nixal_reprap_XidlerComparible_robust (Autodesk Fusion 360 design; units mm, degrees)
Autodesk Fusion 360 part; units mm, degrees
sketch "Sketch1" plane through (0, 0, 0) normal (0, 1, 0) x (1, 0, 0)
  circle A0 centre (0, 0) radius 4
  circle A1 centre (21, -2) radius 4
  circle A2 centre (21, -2) radius 13
  circle A3 centre (21, -2) radius 8 construction
  circle A4 centre (13, -1.9989) radius 1.8
  circle A5 centre (29, -2.0036) radius 1.8
  line L0 (21, -2) -> (21, 11) construction
  line L1 (21, -2) -> (34, -2) construction
  line L2 (41, 31) -> (-24, 31)
  line L3 (41, 31) -> (41, -15)
  circle A6 centre (0, 0) radius 10.5
  circle A7 centre (0, 0) radius 13.5
  line L4 (40.8669, 9) -> (-49.1331, 9)
  line L5 (-49.1331, 9) -> (-49.1331, 26)
  line L6 (-49.1331, 26) -> (40.8669, 26)
  line L7 (40.8669, 26) -> (40.8669, 9)
  line L8 (-13.5, 0) -> (-13.5, 9)
  line L9 (34, -2) -> (34, 9)
  line L10 (0, 0) -> (9.5068, -9.5849)
  line L11 (0, 0) -> (7.6248, -11.8995)
  circle A8 centre (21, -2) radius 5.5
  line L12 (13.3463, 2.0311) -> (12.2858, 9)
  line L13 (9.5068, -9.5849) -> (14.0455, -12.9834)
  circle A9 centre (21, 6) radius 1.8
  circle A10 centre (20.9776, -10) radius 1.8
  circle A11 centre (21, -2) radius 12.6491
  circle A12 centre (0, 0) radius 13.0384
  circle A13 centre (21, -2) radius 5.25
  line L14 (-48.7267, 25.5998) -> (-9.6603, 25.5998)
  line L15 (-9.6603, 25.5998) -> (-9.6603, 9.5175)
  line L16 (-9.6603, 9.5175) -> (-48.7267, 9.5175)
  line L17 (-48.7267, 9.5175) -> (-48.7267, 25.5998)
  line L18 (-9.2762, 9) -> (-9.2762, 26)
  circle A14 centre (0, 0) radius 10.9156
  line L19 (-48.7267, 18.529) -> (-9.6603, 18.529)
  line L20 (-48.7267, 17.955) -> (-9.6603, 17.955)
  circle A15 centre (0, 0) radius 8
  dimension "d1" = 8
  dimension "d2" = 8
  dimension "d23" = 26
  dimension "d104" = 16
  dimension "d107" = 3.6
  dimension "d108" = 3.6
  dimension "d134" = 33
  dimension "d136" = 31
  dimension "d137" = 20
  dimension "d138" = 41
  dimension "d139" = 21
  dimension "d140" = 27
  dimension "d141" = 17
  dimension "d142" = 90
  dimension "d143" = 5
  dimension "d146" = 11
  dimension "d203" = 3.6
  dimension "d204" = 3.6
  dimension "d211" = 90
  dimension "d225" = 10.5
  dimension "d238" = 16
  constraint coincident A0.centre A6.centre
  constraint concentric A1 A2
  constraint coincident A3 A0.centre
  constraint coincident A3
  constraint coincident A2 A0.centre
  constraint vertical L0
  constraint horizontal L1
  constraint horizontal L2
  constraint vertical L3
  constraint concentric A0 A6
  constraint concentric A6 A7
  constraint horizontal L4
  constraint vertical L5
  constraint horizontal L6
  constraint vertical L7
  constraint coincident A7 A0.centre
  constraint coincident L4
  constraint tangent A7 L8
  constraint tangent A2 L9
  constraint coincident A7
  constraint concentric A3 A8
  constraint tangent A7 L12
  constraint coincident A2
  constraint coincident L0 A0.centre
  constraint concentric A1 A11
  constraint concentric A11 A13
  constraint horizontal L14
  constraint vertical L15
  constraint horizontal L16
  constraint vertical L17
  constraint coincident L6
  constraint perpendicular L6 L18
  constraint concentric A12 A14
  constraint coincident L17
  constraint coincident L15
  constraint perpendicular L15 L19
  constraint perpendicular L15 L20
  measures "d1" diameter of A0
  measures "d2" diameter of A1
  measures "d23" diameter of A2
  measures "d104" diameter of A3
  measures "d107" diameter of A4
  measures "d108" diameter of A5
  measures "d134" distance of A0.centre L2
  measures "d136" distance of A0.centre L2
  measures "d137" distance of A0.centre L3
  measures "d138" distance of A0.centre L3
  measures "d139" diameter of A6
  measures "d140" diameter of A7
  measures "d143" distance of L2 L6
  measures "d146" diameter of A8
  measures "d203" diameter of A9
  measures "d204" diameter of A10
  measures "d211" angle of L4 L8
  measures "d225" diameter of A13
  measures "d238" diameter of A15
extrude "Extrude24" add sketch "Sketch1" along normal blind 62 contours A6 L4 L11 A14 | A6 L10 L11 A14 | A2 A6 L10 A14 | A6 L4 A14 | L10 L11 A12 A14 | L4 L11 A12 A14 | A2 A6 A11 A14 | A2 L10 A12 A14 | A2 A6 L4 A14 | L4 A12 L18 A14 | A7 L10 L11 A12 | A7 L4 L11 A12 | A2 A6 A11 A14 | A2 A11 A12 A14 | A6 A11 A14 | A2 A7 L10 A12 | A2 L4 A12 A14 | L4 A12 L18 | A7 L4 A12 L18 | A2 A11 A12 A14 | A2 A7 A11 A12 | A4 A11 A12 A14 | A7 L4 A12 L18 | A2 A7 L4 A12 | A7 L4 L8 | A7 L4 L5 L6 L18 | A2 A7 A11 A12 | A4 A7 A11 A12 | A2 A7 L4 L12 | A2 A7 L4 L6 L7 L18 | A2 A7 L12 A11 | A4 A7 A11 A12 | A4 A7 A12 | A4 A12 | A7 L12 A11 | A2 L4 A11 | L4 A11 | L14 L15 L17 L19 | L15 L17 L19 L20 | L15 L16 L17 L20 makes body 1
extrude "Extrude26" add sketch "Sketch1" along normal blind 62 and the other way blind -54 contours A2 A7 L13 | A2 A7 L4 L13 A11 | A4 A7 L4 L12 A11 | A2 L4 L12 | A2 L4 L12 A11 | A2 L4 L9 bodies 1
sketch "Sketch7" plane through (40.8669, 0, 0) normal (1, 0, 0) x (0, 0, -1)
  line L0 (9, 0) -> (26, 0)
  line L1 (26, 0) -> (26, 62)
  line L2 (26, 62) -> (9, 62)
  line L3 (9, 62) -> (9, 0)
  line L4 (9, 62) -> (26, 0) construction
  line L5 (9, 0) -> (26, 62) construction
  line L6 (17.5, 31) -> (17.5, 53.5) construction
  line L7 (17.5, 31) -> (17.5, 8.5) construction
  circle A0 centre (17.5, 53.5) radius 6
  circle A1 centre (17.5, 8.5) radius 6
  line L8 (23, 46) -> (12, 46)
  line L9 (12, 46) -> (12, 16)
  line L10 (12, 16) -> (23, 16)
  line L11 (23, 16) -> (23, 46)
  line L12 (23, 46) -> (12, 16) construction
  line L13 (12, 46) -> (23, 16) construction
  line L14 (22.7211, 43.5) -> (12.2789, 43.5)
  line L15 (12.2789, 43.5) -> (12.2789, 18.5)
  line L16 (12.2789, 18.5) -> (22.7211, 18.5)
  line L17 (22.7211, 18.5) -> (22.7211, 43.5)
  line L18 (22.7211, 43.5) -> (12.2789, 18.5) construction
  line L19 (12.2789, 43.5) -> (22.7211, 18.5) construction
  line L20 (9, 69.9847) -> (26, 69.9847)
  line L21 (26, 69.9847) -> (26, -8.2428)
  line L22 (26, -8.2428) -> (9, -8.2428)
  line L23 (9, -8.2428) -> (9, 69.9847)
  line L24 (15.7453, 69.9847) -> (18.9725, 69.9847)
  line L25 (18.9725, 69.9847) -> (18.9725, 53.5)
  line L26 (18.9725, 53.5) -> (15.7453, 53.5)
  line L27 (15.7453, 53.5) -> (15.7453, 69.9847)
  line L28 (15.6365, -8.2428) -> (19, -8.2428)
  line L29 (19, -8.2428) -> (19, 8)
  line L30 (19, 8) -> (15.6365, 8)
  line L31 (15.6365, 8) -> (15.6365, -8.2428)
  dimension "d173" = 22.5
  dimension "d174" = 22.5
  dimension "d175" = 12
  dimension "d176" = 12
  dimension "d179" = 30
  dimension "d180" = 11
  dimension "d195" = 25
  constraint midpoint L4
  constraint perpendicular L8 L9
  constraint parallel L8 L10
  constraint parallel L9 L11
  constraint horizontal L8
  constraint coincident L12
  constraint coincident L13
  constraint perpendicular L14 L15
  constraint parallel L14 L16
  constraint parallel L15 L17
  constraint horizontal L14
  constraint coincident L18
  constraint coincident L19
  constraint horizontal L20
  constraint vertical L21
  constraint horizontal L22
  constraint vertical L23
  constraint horizontal L24
  constraint vertical L25
  constraint horizontal L26
  constraint vertical L27
  constraint coincident L20 origin
  constraint horizontal L28
  constraint vertical L29
  constraint horizontal L30
  constraint vertical L31
  constraint coincident L22 origin
  measures "d174" distance of origin
  measures "d175" diameter of A0
  measures "d176" diameter of A1
  measures "d179" distance of origin
  measures "d195" distance of origin
extrude "Extrude27" cut sketch "Sketch7" against normal blind 100 contours A1 L29 L30 L31 | A1 L29 L30 L31 | A0 L25 L26 L27 | A0 L25 L26 L27 bodies 1
extrude "Extrude28" cut sketch "Sketch7" against normal blind 52 contours L8 L9 L10 L11 | L14 L15 L16 L17 bodies 1
sketch "Sketch8" plane through (0, 0, -9) normal (0, 0, 1) x (1, 0, 0)
  line L0 (-49.1331, 0) -> (-13.5, 0)
  line L1 (-13.5, 0) -> (-13.5, 62)
  line L2 (-13.5, 62) -> (-49.1331, 62)
  line L3 (-49.1331, 62) -> (-49.1331, 0)
  line L4 (-49.1331, 62) -> (-13.5, 0) construction
  line L5 (-13.5, 62) -> (-49.1331, 0) construction
  circle A0 centre (-31.3165, 31) radius 15
  line L6 (-15.8165, 47) -> (-46.8165, 47) construction
  line L7 (-46.8165, 47) -> (-46.8165, 15) construction
  line L8 (-46.8165, 15) -> (-15.8165, 15) construction
  line L9 (-15.8165, 15) -> (-15.8165, 47) construction
  line L10 (-15.8165, 47) -> (-46.8165, 15) construction
  line L11 (-46.8165, 47) -> (-15.8165, 15) construction
  circle A1 centre (-46.8165, 47) radius 1.65
  circle A2 centre (-15.8165, 47) radius 1.65
  circle A3 centre (-46.8165, 15) radius 1.65
  circle A4 centre (-15.8165, 15) radius 1.65
  circle A5 centre (-46.8165, 47) radius 3
  circle A6 centre (-15.8165, 47) radius 3
  circle A7 centre (-15.8165, 15) radius 3
  line L12 (-49.1331, 38.5778) -> (-44.2617, 38.5778)
  line L13 (-24.2799, 0) -> (-24.2799, 17.7529)
  line L14 (-49.1331, 62) -> (-13.5, 62)
  line L15 (-13.5, 62) -> (-13.5, 0)
  line L16 (-13.5, 0) -> (-49.1331, 0)
  line L17 (-49.1331, 0) -> (-49.1331, 62)
  arc A8 (-44.1331, 62) -> (-49.1331, 57) centre (-44.1331, 57) ccw
  line L18 (-49.1331, 62) -> (-13.5, 62)
  line L19 (-13.5, 62) -> (-13.5, 70.2436)
  line L20 (-13.5, 70.2436) -> (-49.1331, 70.2436)
  line L21 (-49.1331, 70.2436) -> (-49.1331, 62)
  dimension "d183" = 30
  dimension "d184" = 31
  dimension "d185" = 32
  dimension "d186" = 3.3
  dimension "d187" = 3.3
  dimension "d188" = 3.3
  dimension "d189" = 3.3
  dimension "d190" = 6
  dimension "d191" = 6
  dimension "d192" = 6
  dimension "d202" = 5
  constraint midpoint L4
  constraint perpendicular L6 L7
  constraint parallel L6 L8
  constraint parallel L7 L9
  constraint horizontal L6
  constraint coincident L10
  constraint coincident L11
  constraint concentric A1 A5
  constraint coincident L3 origin
  constraint perpendicular L7 L12
  constraint coincident A0 origin
  constraint perpendicular L8 L13
  constraint horizontal L14
  constraint vertical L15
  constraint horizontal L16
  constraint vertical L17
  constraint coincident L16 origin
  constraint tangent L14 A8
  constraint tangent L17 A8
  constraint coincident L14
  constraint coincident L17
  constraint horizontal L18
  constraint vertical L19
  constraint horizontal L20
  constraint vertical L21
  measures "d183" diameter of A0
  measures "d184" distance of origin
  measures "d186" diameter of A1
  measures "d187" diameter of A2
  measures "d188" diameter of A3
  measures "d189" diameter of A4
  measures "d190" diameter of A5
  measures "d191" diameter of A6
  measures "d192" diameter of A7
  measures "d202" radius of A8
extrude "Extrude29" cut sketch "Sketch8" against normal blind 40 contours L0 L3 A0 L12 L13 L16 L17 | A0 | L2 L3 L14 L17 A8 L18 | A3 bodies 1
extrude "Extrude30" cut sketch "Sketch7" against normal blind 65 contours L14 L15 L16 L17 bodies 1
extrude "Extrude31" cut sketch "Sketch8" against normal blind 40 contours A1 | A2 | A4 bodies 1
extrude "Extrude32" cut sketch "Sketch8" against normal blind 9 contours L3 A5 L17 | L3 A5 L17 | L1 A7 L15 | L1 A7 L15 | L1 A6 L15 | L1 A6 L15 bodies 1
extrude "Extrude33" add sketch "Sketch7" against normal blind 50 contours L0 L22 L23 L31 | L0 L22 L28 L29 L31 | L2 L20 L23 L27 | L0 L21 L22 L29 | L2 L20 L24 L25 L27 | L2 L20 L21 L25 bodies 1
extrude "Extrude34" cut sketch "Sketch7" against normal blind 50 contours L2 L20 L24 L25 L27 | L2 A0 L25 L27 | A0 L25 L26 L27 picked at (17.3571, 55.4994) bodies 1
extrude "Extrude35" cut sketch "Sketch7" against normal blind 50 contours L0 A1 L29 L31 | L0 L22 L28 L29 L31 | A1 L29 L30 L31 picked at (17.3157, 6.1677) bodies 1
extrude "Extrude36" cut sketch "Sketch1" along normal blind 65 contours A6 L10 L11 A14 | L10 L11 A12 A14 | A7 L10 L11 A12 bodies 1
sketch "Sketch9" plane through (0, -8.2428, 0) normal (0, -1, 0) x (1, 0, 0)
  line L0 (-9.1331, -15.6365) -> (40.8669, -15.6365)
  line L1 (40.8669, -15.6365) -> (40.8669, -9)
  line L2 (40.8669, -9) -> (-9.1331, -9)
  line L3 (-9.1331, -9) -> (-9.1331, -15.6365)
  circle A0 centre (0, 0) radius 10.5
  line L4 (40.8669, -9) -> (-49.1331, -9)
extrude "Extrude37" cut sketch "Sketch9" against normal blind 80 contours L2 A0 L4 picked at (1.3817, -9.2157) bodies 1
sketch "Sketch10" plane through (0, 0, -26) normal (0, 0, -1) x (-1, 0, 0)
  circle A0 centre (46.8165, 47) radius 1.65
  circle A1 centre (15.8165, 47) radius 1.65
  circle A2 centre (15.8165, 15) radius 1.65
  arc A3 (49.1331, 57) -> (44.1331, 62) centre (44.1331, 57) ccw
  line L0 (44.1331, 62) -> (9.1331, 62)
  line L1 (9.1331, 62) -> (9.1331, 69.9847)
  line L2 (9.1331, 69.9847) -> (-40.8669, 69.9847)
  line L3 (-40.8669, 69.9847) -> (-40.8669, -8.2428)
  line L4 (-40.8669, -8.2428) -> (9.1331, -8.2428)
  line L5 (9.1331, -8.2428) -> (9.1331, 0)
  line L6 (9.1331, 0) -> (24.2799, 0)
  line L7 (24.2799, 0) -> (24.2799, 17.7529)
  arc A4 (44.2617, 38.5778) -> (24.2799, 17.7529) centre (31.3165, 31) ccw
  line L8 (44.2617, 38.5778) -> (49.1331, 38.5778)
  line L9 (49.1331, 38.5778) -> (49.1331, 57)
  circle A5 centre (-35, 66) radius 1.65
  circle A6 centre (-11, 66) radius 1.65
  circle A7 centre (-11, -4) radius 1.65
  circle A8 centre (-35, -4) radius 1.65
  dimension "d216" = 3.3
  dimension "d217" = 3.3
  dimension "d220" = 3.3
  dimension "d221" = 3.3
  measures "d216" diameter of A5
  measures "d217" diameter of A6
  measures "d220" diameter of A7
  measures "d221" diameter of A8
extrude "Extrude38" cut sketch "Sketch10" against normal blind 31 contours A5 | A6 | A7 | A8 bodies 1
extrude "Extrude39" add sketch "Sketch1" along normal blind 70 and the other way blind -62 separate body contours A7 L10 L11 A12 | A7 L4 L11 A12 | A2 A7 L13 | A2 A7 L4 L13 A11 makes body 2
extrude "Extrude40" add sketch "Sketch1" along normal blind 70 and the other way blind -62 separate body contours A8 makes body 3
extrude "Extrude41" add sketch "Sketch1" along normal blind 70 and the other way blind -62 separate body contours A7 L4 L5 L6 L18 makes body 4
extrude "Extrude42" add sketch "Sketch1" along normal blind 70 and the other way blind -62 separate body contours A6 L4 L11 A14 | A6 L10 L11 A14 | A2 A6 L10 A14 | A6 L4 A14 | A2 A6 A11 A14 | A2 A6 L4 A14 | A2 A6 A11 A14 | A6 A11 A14 makes body 5
extrude "Extrude43" add sketch "Sketch1" along normal blind 70 and the other way blind -62 separate body contours L15 L17 L19 L20 makes body 6
extrude "Extrude44" add sketch "Sketch1" along normal blind 62 contours A2 A6 L4 L10 L11 A15 | A2 A6 A11 | A6 A11 bodies 1 5
extrude "Extrude45" cut sketch "Sketch8" against normal blind 85 contours L0 L1 L2 L3 A0 A5 A6 A7 L12 L13 L14 L15 L16 L17 A8 L18 | L3 A5 L17 | L1 A7 L15 | L1 A6 L15 | L2 L14 L18 L19 L20 L21 picked at (-48.9109, 47) picked at (-13.7222, 15) picked at (-13.7222, 47) bodies 1 4 6
equation "d173 = ( 45 / 2 ) * 1 mm"
equation "d174 = ( 45 / 2 ) * 1 mm"
